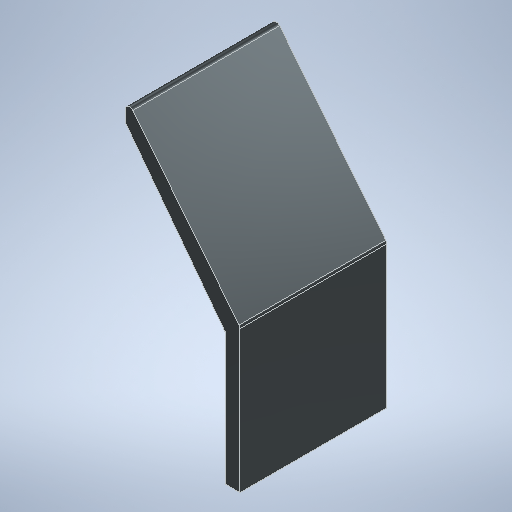
# Autodesk Inventor part: mechanism
Saved by Autodesk Inventor 2025.1 (Build 291241000, 241)
## iProperties
Created: 2024-10-22
Part Number: mechanism
Material: Iron, Ductile
Document SubType Name: Modeling
Designer: vedan
Density: 7.15 g/cm^3
Appearance: Iron Gray
Author: vedan
Autodesk Inventor part; units mm, degrees
ref_plane "YZ Plane" through (0, 0, 0) normal (1, 0, 0) x (0, 1, 0)
ref_plane "XZ Plane" through (0, 0, 0) normal (0, 1, 0) x (-1, 0, 0)
ref_plane "XY Plane" through (0, 0, 0) normal (0, 0, 1) x (1, 0, 0)
sketch "Sketch1" plane through (0, 0, 0) normal (1, 0, 0) x (0, 1, 0)
  line L0 (0, 0) -> (100, 0)
  line L1 (100, 0) -> (100, -102.3)
  line L2 (100, -102.3) -> (0, -102.3)
  line L3 (0, -102.3) -> (0, 0)
  dimension "d0" = 102.3
  dimension "d1" = 100
  constraints: 8 end point, 2 parallel, 1 horizontal, 1 perpendicular
  measures "d0" distance of L2.end L0.start
  measures "d1" distance of L1.end L2.end
extrude "Extrusion1" add sketch "Sketch1" along normal blind 80
sketch "Sketch3" plane through (0, 0, 0) normal (0, 0, 1) x (1, 0, 0)
  line L0 (0, 100) -> (0, 200)
  line L1 (0, 200) -> (80, 100)
  line L2 (0, 100) -> (80, 100)
  dimension "d4" = 100
  dimension "d8" = 128.0625
  dimension "d15" = 80
  constraints: 6 end point, 1 horizontal, 1 vertical
  measures "d4" distance of L0.start L0.end
  measures "d8" distance of L0.end L1.end
  measures "d15" distance of L0.start L1.end
extrude "Extrusion2" add sketch "Sketch3" against normal blind 102.3
sketch "Sketch8" plane through (0, 0, 0) normal (0, 0, 1) x (1, 0, 0)
  line L0 (0, 0) -> (80, 0) projected
  line L1 (80, 100) -> (0, 200) projected
  line L2 (0, 183.4727) -> (0, 0)
  line L3 (0, 0) -> (62.6268, 0)
  line L4 (0, 183.4727) -> (69.6704, 91.7363)
  line L5 (69.6704, 91.7363) -> (69.6704, 0)
  line L6 (0, 183.4727) -> (0, 200)
  line L7 (0, 200) -> (80, 100)
  line L8 (80, 100) -> (80, 0)
  line L9 (69.6704, 0) -> (80, 0)
  constraints: 16 end point, 3 vertical, 2 horizontal, 1 perpendicular, 1 point on line
extrude "Extrusion5" cut sketch "Sketch8" against normal through all contours L2 L4 L5 L0
fillet "Fillet2" radius 3 2 edges at (0, 200, -51.15) (80, 100, -51.15)
sketch "Sketch9" plane through (80, 0, -102.3) normal (0, -1, 0) x (1, 0, 0)
  line L0 (-6.3296, 95.6) -> (-6.3296, 102.3) construction
  line L1 (-80, 102.3) -> (0, 102.3) construction
  line L2 (-6.3296, 6.7) -> (-6.3296, 0) construction
  line L3 (-10.3296, 0) -> (0, 0) construction
  line L4 (-10.3296, 102.3) -> (-10.3296, 0) projected
  point P0 (-80, 0)
  dimension "d43" = 88.9
  dimension "d44" = 6.7
  dimension "d53" = 4
  constraints: 4 end point, 2 point on line, 2 vertical, 1 vertical alignment
  measures "d43" distance of L2.start L0.start
  measures "d44" distance of L0.end L0.start
  measures "d53" distance from line of L0.start L4
hole "Hole3" at (73.6704, 0, -6.7) at (73.6704, 0, -95.6) direction (0, 1, 0) diameter 4.25 depth 8 tip angle 118
body "Solid1"
